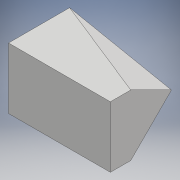
# Autodesk Inventor part: 40
Saved by Autodesk Inventor 2017 (Build 210142000, 142)
## iProperties
Part Number: 40
Material: 一般
Document SubType Name: Modeling
Designer: Brian
Density: 1 g/cm^3
Appearance: 預設
Author: Brian
Autodesk Inventor part; units mm, degrees
ref_plane "YZ Plane" through (0, 0, 0) normal (1, 0, 0) x (0, 1, 0)
sketch "草圖1" plane through (0, 0, 0) normal (0, 1, 0) x (-1, 0, 0)
  line L0 (0, 0) -> (-50, 0)
  line L1 (-50, 0) -> (-50, -30)
  line L2 (-50, -30) -> (0, -30)
  line L3 (0, -30) -> (0, 0)
  dimension "d0" = 30
  dimension "d1" = 50
  constraints: 8 end point, 2 parallel, 1 horizontal, 1 perpendicular
  measures "d0" distance of L2.end L0.start
  measures "d1" distance of L1.end L2.end
extrude "擠出1" add sketch "草圖1" along normal blind 30
sketch "草圖2" plane through (50, 0, 0) normal (1, 0, 0) x (0, 0, -1)
  line L0 (0, 0) -> (0, 30) projected
  line L1 (0, 10) -> (10, 30)
  line L2 (0, 30) -> (30, 30) projected
  dimension "d4" = 10
  dimension "d5" = 20
  constraints: 2 end point, 2 point on line
  measures "d4" horizontal distance of L1.start L1.end
  measures "d5" vertical distance of L1.start L1.end
ref_plane "工作平面1" through (0, 30, 0) normal (0.1761, 0.4402, 0.8805) x (0.9285, -0.3714, 0)
sketch "草圖3" plane through (0, 30, 0) normal (0.1761, 0.4402, 0.8805) x (0.9285, -0.3714, 0)
  line L0 (-15.4491, 27.3305) -> (88.7028, 27.3305)
  line L1 (88.7028, 27.3305) -> (88.7028, -20.9863)
  line L2 (88.7028, -20.9863) -> (-15.4491, -20.9863)
  line L3 (-15.4491, -20.9863) -> (-15.4491, 27.3305)
  point P0 (11.1417, -24.5243)
  constraints: 8 end point, 2 parallel, 1 horizontal, 1 perpendicular
extrude "擠出2" cut sketch "草圖3" along normal blind 30
sketch "草圖4" plane through (50, 0, 0) normal (1, 0, 0) x (0, 0, -1)
  line L0 (30, 0) -> (30, 30) projected
  point P0 (0, 0)
  point P1 (30, 10)
  dimension "d8" = 20
  constraints: 1 point on line
  measures "d8" distance of L0.end point (30, 10)
ref_plane "工作平面2" through (0, 30, -30) normal (0.2722, 0.6804, -0.6804) x (0.9285, 0, 0.3714)
sketch "草圖5" plane through (0, 30, -30) normal (0.2722, 0.6804, -0.6804) x (0.9285, 0, 0.3714)
  line L0 (63.1624, -12.2255) -> (-24.2943, -12.2255)
  line L1 (-24.2943, -12.2255) -> (-24.2943, 28.5728)
  line L2 (-24.2943, 28.5728) -> (63.1624, 28.5728)
  line L3 (63.1624, 28.5728) -> (63.1624, -12.2255)
  point P0 (11.1417, 3.0324)
  constraints: 8 end point, 2 parallel, 1 horizontal, 1 perpendicular
extrude "擠出3" cut sketch "草圖5" along normal blind 30
